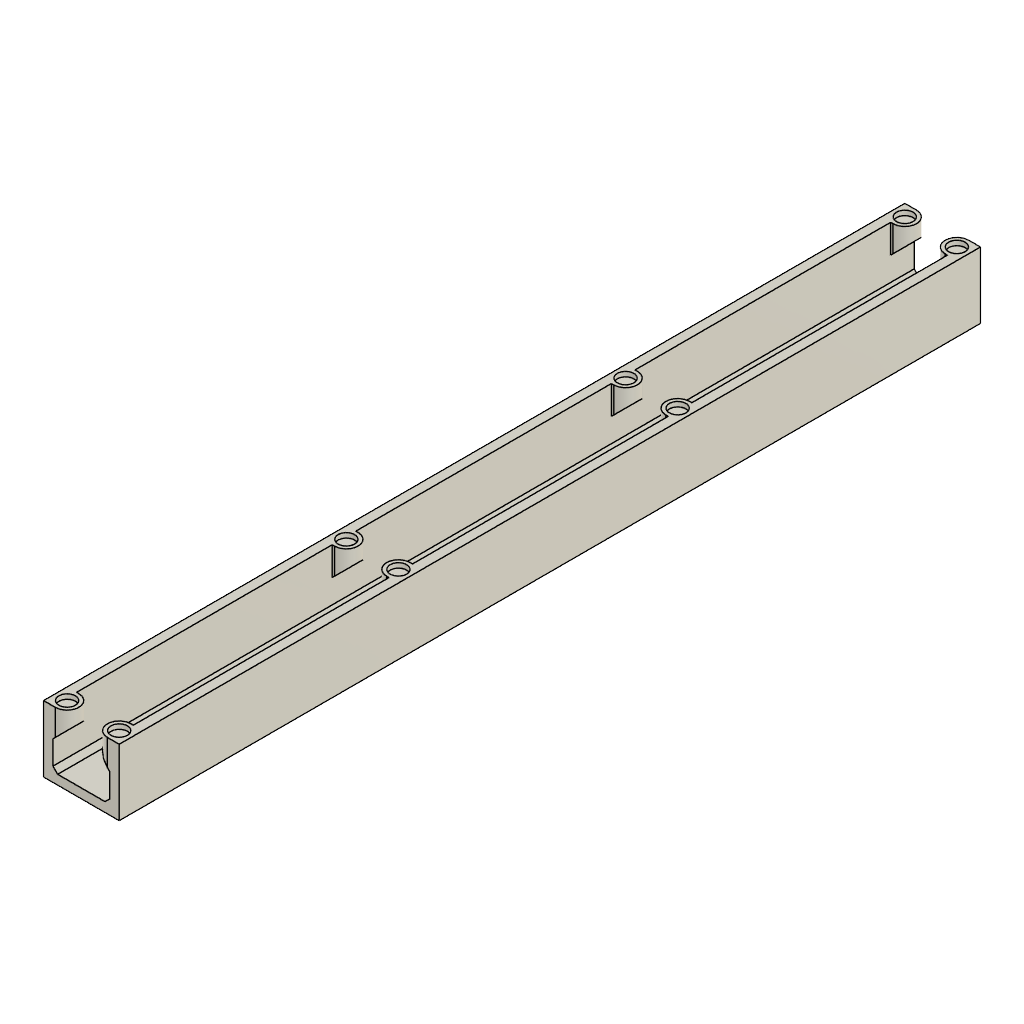
lower_wire_management_conduit (Autodesk Fusion 360 archive; units mm, degrees)
design "Lower Wire Management Conduit Bottom"
part number: 2026-09-19-14-55-36-645
Autodesk Fusion 360 part; units mm, degrees
note: some values were not read from the file. Set by a fixed rule: which sketch regions a step uses.
sketch "3D-printed conduit outline" plane through (0, 0, 0) normal (0, 1, 0) x (1, 0, 0)
  line L0 (0, 0) -> (16, 0)
  line L1 (16, 0) -> (16, -14)
  line L2 (16, -14) -> (0, -14)
  line L3 (0, -14) -> (0, 0)
  line L4 (2, -14) -> (14, -14)
  line L5 (14, -14) -> (14, -2)
  line L6 (14, -2) -> (2, -2)
  line L7 (2, -2) -> (2, -14)
  dimension "d8" = 14
  dimension "d9" = 16
  dimension "d10" = 2
  dimension "d11" = 2
  dimension "d12" = 2
  constraint horizontal L0
  constraint vertical L1
  constraint horizontal L2
  constraint vertical L3
  constraint coincident L0.start L3.end
  constraint horizontal L4
  constraint vertical L5
  constraint horizontal L6
  constraint vertical L7
  constraint coincident L2 L4.start
  measures "d8" distance of L0.start L2.end
  measures "d9" distance of L0.start L0.end
  measures "d10" distance of L1 L5
  measures "d11" distance of L3 L7
  measures "d12" distance of L0 L6
extrude "Extrude1" add sketch "3D-printed conduit outline" along normal blind 182 contours L0 L1 L2 L3 L5 L6 L7
sketch "Magnet holders" plane through (0, 0, 14) normal (0, 0, 1) x (-1, 0, 0)
  line L0 (0, 0) -> (-2, 0)
  line L1 (-2, 0) -> (-2, -182)
  line L2 (-2, -182) -> (0, -182)
  line L3 (0, -182) -> (0, 0)
  line L4 (-14, 0) -> (-16, 0)
  line L5 (-16, 0) -> (-16, -182)
  line L6 (-16, -182) -> (-14, -182)
  line L7 (-14, -182) -> (-14, 0)
  circle A0 centre (-2.5, -2.5) radius 2.5
  circle A1 centre (-2.5, -2.5) radius 1.75
  line L8 (-14, 0) -> (-2, 0)
  line L9 (0, 0) -> (-2.5, 0)
  line L10 (-2.5, 0) -> (-2.5, -5)
  line L11 (-2.5, -5) -> (0, -5)
  line L12 (0, -5) -> (0, 0)
  circle A2 centre (-13.5, -2.5) radius 2.5
  circle A3 centre (-13.5, -2.5) radius 1.75
  line L13 (-16, 0) -> (-13.5, 0)
  line L14 (-13.5, 0) -> (-13.5, -5)
  line L15 (-13.5, -5) -> (-16, -5)
  line L16 (-16, -5) -> (-16, 0)
  circle A4 centre (-2.5, -61.5) radius 1.75
  circle A5 centre (-2.5, -61.5) radius 2.5
  line L17 (-2.5, -59) -> (-2.5, -64)
  line L18 (-2.5, -64) -> (0, -64)
  line L19 (0, -64) -> (0, -59)
  line L20 (0, -59) -> (-2.5, -59)
  circle A6 centre (-13.5, -61.5) radius 1.75
  circle A7 centre (-13.5, -61.5) radius 2.5
  line L21 (-13.5, -59) -> (-13.5, -64)
  line L22 (-13.5, -64) -> (-16, -64)
  line L23 (-16, -64) -> (-16, -59)
  line L24 (-16, -59) -> (-13.5, -59)
  circle A8 centre (-2.5, -120.5) radius 1.75
  circle A9 centre (-2.5, -120.5) radius 2.5
  line L25 (-2.5, -118) -> (-2.5, -123)
  line L26 (-2.5, -123) -> (0, -123)
  line L27 (0, -123) -> (0, -118)
  line L28 (0, -118) -> (-2.5, -118)
  circle A10 centre (-13.5, -120.5) radius 1.75
  circle A11 centre (-13.5, -120.5) radius 2.5
  line L29 (-13.5, -118) -> (-13.5, -123)
  line L30 (-13.5, -123) -> (-16, -123)
  line L31 (-16, -123) -> (-16, -118)
  line L32 (-16, -118) -> (-13.5, -118)
  circle A12 centre (-2.5, -179.5) radius 1.75
  circle A13 centre (-2.5, -179.5) radius 2.5
  line L33 (-2.5, -177) -> (-2.5, -182)
  line L34 (-2.5, -182) -> (0, -182)
  line L35 (0, -182) -> (0, -177)
  line L36 (0, -177) -> (-2.5, -177)
  circle A14 centre (-13.5, -179.5) radius 1.75
  circle A15 centre (-13.5, -179.5) radius 2.5
  line L37 (-13.5, -177) -> (-13.5, -182)
  line L38 (-13.5, -182) -> (-16, -182)
  line L39 (-16, -182) -> (-16, -177)
  line L40 (-16, -177) -> (-13.5, -177)
  dimension "d15" = 5
  dimension "d16" = 3.5
  dimension "d17" = 5
  dimension "d18" = 3.5
  dimension "d21" = 0
  dimension "d22" = -177
  constraint concentric A0 A1
  constraint tangent A0 L8
  constraint tangent L3 A0
  constraint horizontal L9
  constraint vertical L10
  constraint horizontal L11
  constraint vertical L12
  constraint coincident L0.start L3.end
  constraint tangent A0 L11
  constraint coincident A0 L9.end
  constraint concentric A2 A3
  constraint tangent L5 A2
  constraint tangent L8 A2
  constraint horizontal L13
  constraint vertical L14
  constraint horizontal L15
  constraint vertical L16
  constraint coincident L4.end L5.start
  constraint tangent A2 L15
  constraint coincident A2 L13.end
  measures "d15" diameter of A0
  measures "d16" diameter of A1
  measures "d17" diameter of A2
  measures "d18" diameter of A3
extrude "Extrude2" add sketch "Magnet holders" against normal blind 3 contours L1 A0 L8 L9 | L1 A0 A1 L10 | A0 A1 L10 | L1 A0 A1 L10 | L1 A0 L11 | L1 A1 L10 | A1 L10 | L1 A5 L20 | L1 A4 A5 L17 | L1 A4 A5 L17 | L1 A5 L18 | A4 A5 L17 | L1 A4 L17 | A4 L17 | L1 A9 L28 | L1 A8 A9 L25 | L1 A8 A9 L25 | L1 A9 L26 | A8 A9 L25 | L1 A8 L25 | A8 L25 | L1 A13 L36 | L1 A12 A13 L33 | L1 A12 A13 L33 | L1 A13 L34 | A12 A13 L33 | L1 A12 L33 | A12 L33 | L7 L8 A2 L13 | L7 A2 A3 L14 | A2 A3 L14 | L7 A3 L14 | A3 L14 | L7 A2 L15 | L7 A2 A3 L14 | L7 A7 L24 | L7 A6 A7 L21 | L7 A7 L22 | L7 A6 A7 L21 | A6 A7 L21 | L7 A6 L21 | A6 L21 | L7 A11 L32 | L7 A10 A11 L29 | L7 A11 L30 | L7 A10 A11 L29 | A10 A11 L29 | L7 A10 L29 | A10 L29 | L7 A15 L40 | L7 A14 A15 L37 | L7 A15 L38 | L7 A14 A15 L37 | A14 A15 L37 | L7 A14 L37 | A14 L37
extrude "Extrude3" cut sketch "Magnet holders" against normal blind 1 contours L1 A1 | L1 A1 L10 | A1 L10 | L1 A4 | L1 A4 L17 | A4 L17 | L1 A8 | L1 A8 L25 | A8 L25 | L1 A12 | L1 A12 L33 | A12 L33 | L7 A3 L14 | L7 A3 | A3 L14 | L7 A6 L21 | L7 A6 | A6 L21 | L7 A10 L29 | L7 A10 | A10 L29 | L7 A14 L37 | L7 A14 | A14 L37
chamfer "Chamfer1" distance 1 angle 45 2 edges at (2, 91, 2) (14, 91, 2)
chamfer "Chamfer2" distance 2.9999 angle 45 8 edges at (2, 2.5, 11) (2, 61.5, 11) (2, 120.5, 11) (2, 179.5, 11) (14, 2.5, 11) (14, 61.5, 11) (14, 120.5, 11) (14, 179.5, 11)
equation "conduit_length = 182.00 mm"
equation "conduit_width = 16 mm"
equation "conduit_height = 16 mm"
equation "conduit_wall_thickness = 2 mm"
equation "magnet_diameter = 3 mm"
equation "magnet_height = 1 mm"
equation "number_of_magnets_on_a_side = 4"
equation "d8 = conduit_height - conduit_wall_thickness"
equation "d9 = conduit_width"
equation "d10 = conduit_wall_thickness"
equation "d11 = conduit_wall_thickness"
equation "d12 = conduit_wall_thickness"
equation "d13 = conduit_length"
equation "d15 = magnet_diameter + 2 mm"
equation "d16 = magnet_diameter + 0.5 mm"
equation "d17 = magnet_diameter + 2 mm"
equation "d18 = magnet_diameter + 0.5 mm"
equation "d20 = number_of_magnets_on_a_side"
equation "d22 = -conduit_length + ( magnet_diameter + 2 mm )"
equation "d23 = -( magnet_height + 2 mm )"
equation "d25 = -magnet_height"
named bodies: "Lower wire management conduit bottom"

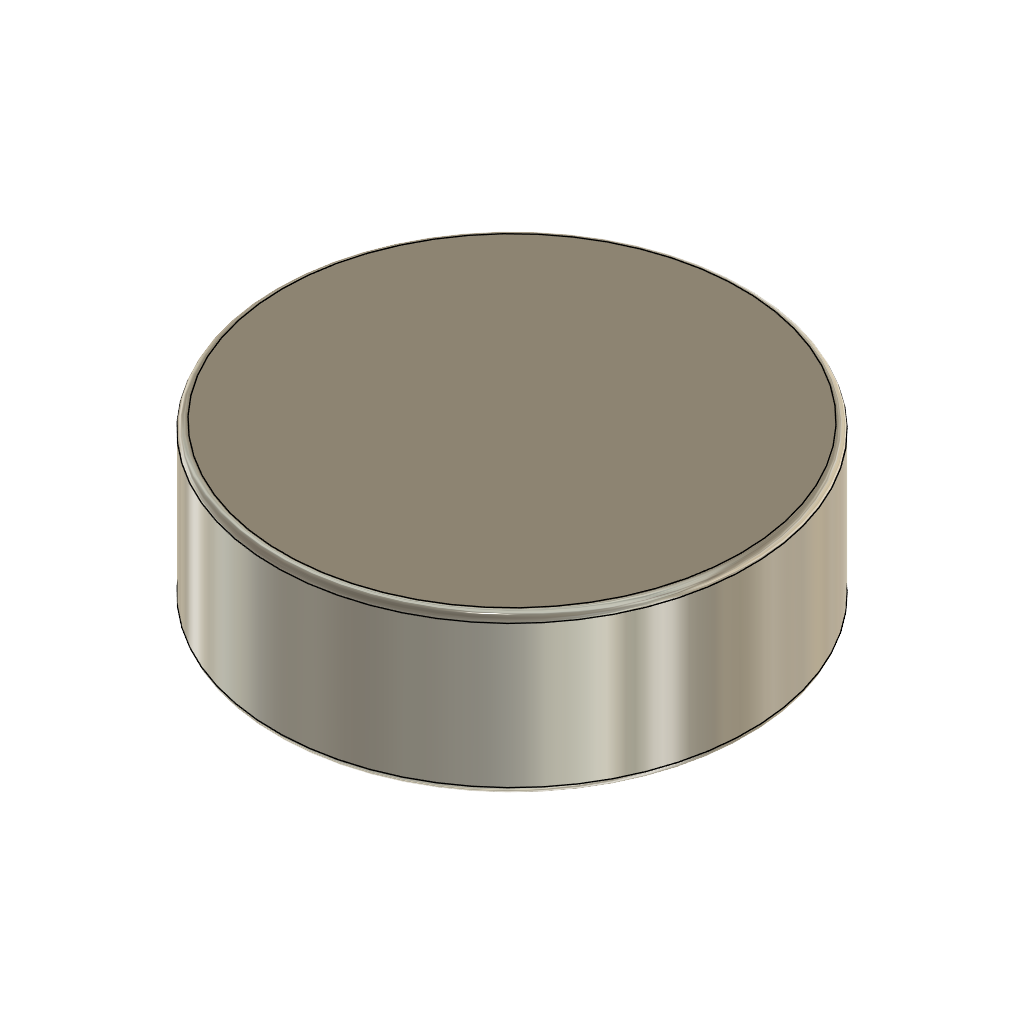
design "3 mm x 1 mm Neodymium Disc Magnet"
Autodesk Fusion 360 part; units mm, degrees
sketch "3 mm x 1 mm neodymium disc magnet" plane through (0, 0, 0) normal (0, 0, 1) x (1, 0, 0)
  circle A0 centre (0, 0) radius 1.5
  dimension "d1" = 3
  constraint coincident A0.centre origin
  measures "d1" diameter of A0
extrude "Extrude1" add sketch "3 mm x 1 mm neodymium disc magnet" along normal blind 1
fillet "Fillet1" radius 0.05 2 edges at (-1.3985, -0.5424, 1) (-1.3985, -0.5424, 0)
named bodies: "3 mm x 1 mm Neodymium Disc Magnet"

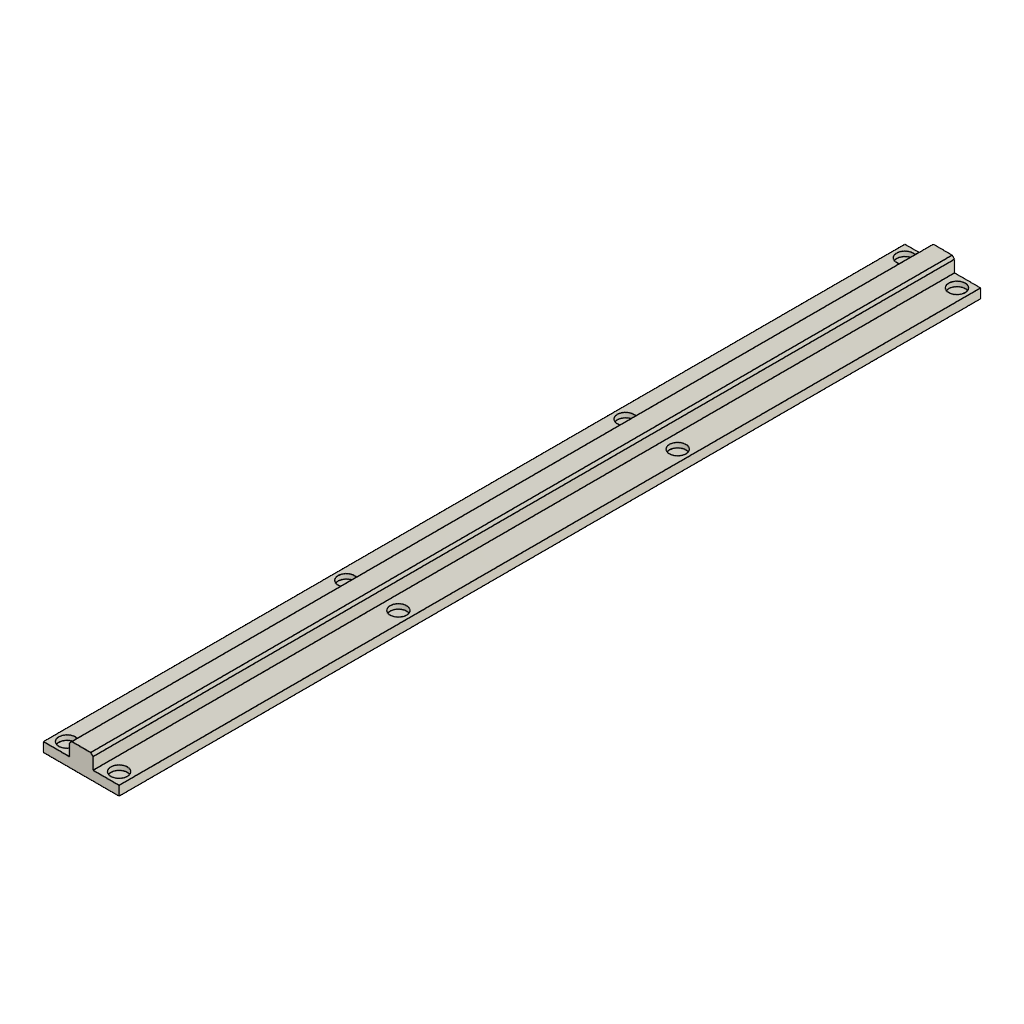
design "Lower Wire Management Conduit Top"
part number: 2026-09-19-15-15-46-900
Autodesk Fusion 360 part; units mm, degrees
sketch "3D-printed conduit top outline" plane through (0, 0, 0) normal (0, 1, 0) x (1, 0, 0)
  line L0 (0, 0) -> (16, 0)
  line L1 (16, 0) -> (16, -2)
  line L2 (16, -2) -> (0, -2)
  line L3 (0, -2) -> (0, 0)
  dimension "d7" = 16
  dimension "d8" = 2
  constraint horizontal L0
  constraint vertical L1
  constraint horizontal L2
  constraint vertical L3
  constraint coincident L0.start L3.end
  measures "d7" distance of L0.start L0.end
  measures "d8" distance of L0.start L2.end
extrude "Extrude1" add sketch "3D-printed conduit top outline" along normal blind 182
sketch "Magnet holes" plane through (0, 0, 2) normal (0, 0, 1) x (-1, 0, 0)
  line L0 (0, 0) -> (-16, 0)
  line L1 (-16, 0) -> (-16, -182)
  line L2 (-16, -182) -> (0, -182)
  line L3 (0, -182) -> (0, 0)
  circle A0 centre (-2.5, -2.5) radius 2.5
  circle A1 centre (-13.5, -2.5) radius 2.5
  circle A2 centre (-2.5, -2.5) radius 1.75
  circle A3 centre (-13.5, -2.5) radius 1.75
  circle A4 centre (-2.5, -61.5) radius 1.75
  circle A5 centre (-2.5, -61.5) radius 2.5
  circle A6 centre (-13.5, -61.5) radius 2.5
  circle A7 centre (-13.5, -61.5) radius 1.75
  circle A8 centre (-2.5, -120.5) radius 1.75
  circle A9 centre (-2.5, -120.5) radius 2.5
  circle A10 centre (-13.5, -120.5) radius 2.5
  circle A11 centre (-13.5, -120.5) radius 1.75
  circle A12 centre (-2.5, -179.5) radius 1.75
  circle A13 centre (-2.5, -179.5) radius 2.5
  circle A14 centre (-13.5, -179.5) radius 2.5
  circle A15 centre (-13.5, -179.5) radius 1.75
  dimension "d11" = 5
  dimension "d12" = 5
  dimension "d13" = 3.5
  dimension "d14" = 3.5
  dimension "d17" = 0
  dimension "d18" = -177
  constraint concentric A0 A2
  constraint concentric A1 A3
  constraint tangent L3 A0
  constraint tangent L0 A0
  constraint tangent L1 A1
  constraint tangent L0 A1
  measures "d11" diameter of A0
  measures "d12" diameter of A1
  measures "d13" diameter of A2
  measures "d14" diameter of A3
extrude "Extrude2" cut sketch "Magnet holes" against normal blind 1 contours A2 | A3 | A4 | A7 | A8 | A11 | A12 | A15
sketch "Support rib" plane through (0, 0, 2) normal (0, 0, 1) x (-1, 0, 0)
  line L0 (0, 0) -> (-16, 0)
  line L1 (-16, 0) -> (-16, -182)
  line L2 (-16, -182) -> (0, -182)
  line L3 (0, -182) -> (0, 0)
  circle A0 centre (-13.5, -179.5) radius 1.75
  circle A1 centre (-13.5, -61.5) radius 1.75
  circle A2 centre (-2.5, -2.5) radius 1.75
  circle A3 centre (-2.5, -120.5) radius 1.75
  circle A4 centre (-2.5, -179.5) radius 1.75
  circle A5 centre (-2.5, -61.5) radius 1.75
  circle A6 centre (-13.5, -2.5) radius 1.75
  circle A7 centre (-13.5, -120.5) radius 1.75
  line L4 (-5.5, 0) -> (-10.5, 0)
  line L5 (-10.5, 0) -> (-10.5, -182)
  line L6 (-10.5, -182) -> (-5.5, -182)
  line L7 (-5.5, -182) -> (-5.5, 0)
  dimension "d23" = 5
  dimension "d24" = 5.5
  dimension "d25" = 5.5
  constraint horizontal L4
  constraint vertical L5
  constraint horizontal L6
  constraint vertical L7
  constraint coincident L2 L5.end
  constraint coincident L0 L4.start
  measures "d23" distance of L5 L7
  measures "d24" distance of L3 L7
  measures "d25" distance of L1 L5
extrude "Extrude3" add sketch "Support rib" along normal blind 3 contours L0 L2 L4 L5 L6 L7
chamfer "Chamfer1" distance 0.5 angle 45 2 edges at (5.5, 91, 5) (10.5, 91, 5)
equation "conduit_length = 182.00 mm"
equation "conduit_width = 16 mm"
equation "conduit_wall_thickness = 2 mm"
equation "magnet_diameter = 3 mm"
equation "magnet_height = 1 mm"
equation "number_of_magnets_on_a_side = 4"
equation "d7 = conduit_width"
equation "d8 = conduit_wall_thickness"
equation "d9 = conduit_length"
equation "d11 = magnet_diameter + 2 mm"
equation "d12 = magnet_diameter + 2 mm"
equation "d13 = magnet_diameter + 0.5 mm"
equation "d14 = magnet_diameter + 0.5 mm"
equation "d16 = number_of_magnets_on_a_side"
equation "d18 = -conduit_length + magnet_diameter + 2 mm"
equation "d19 = -magnet_height"
equation "rib_width = 5 mm"
equation "rib_height = 3 mm"
equation "d23 = rib_width"
equation "d24 = ( conduit_width - rib_width ) / 2"
equation "d26 = rib_height"
equation "rib_chamfer = 0.5 mm"
equation "d29 = rib_chamfer"
named bodies: "Lower wire management conduit top"
